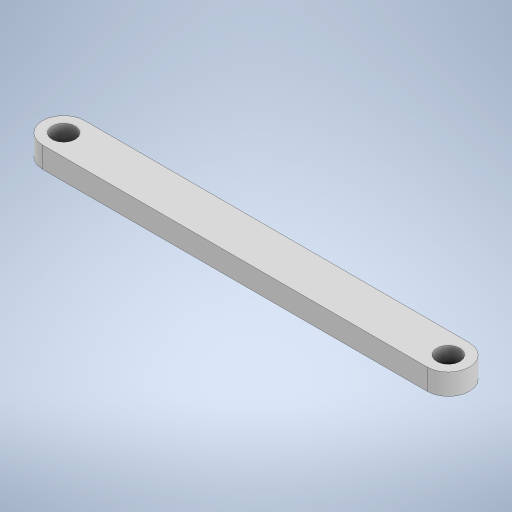
# Autodesk Inventor part: connector
Saved by Autodesk Inventor 2024 (Build 280153000, 153)
## iProperties
Created: 2024-03-19
Part Number: connector
Material: Generic
Document SubType Name: Modeling
Designer: maja6
Density: 1 g/cm^3
Appearance: Default
Author: maja6
Autodesk Inventor part; units mm, degrees
ref_plane "YZ Plane" through (0, 0, 0) normal (1, 0, 0) x (0, 1, 0)
ref_plane "XZ Plane" through (0, 0, 0) normal (0, 1, 0) x (-1, 0, 0)
ref_plane "XY Plane" through (0, 0, 0) normal (0, 0, 1) x (1, 0, 0)
sketch "Sketch1" plane through (0, 0, 0) normal (0, 0, 1) x (1, 0, 0)
  line L0 (0, 0) -> (24, 0)
  circle A0 centre (0, 0) radius 1.6
  line L1 (0, 0) -> (24, 0) construction
  line L2 (0, -3) -> (24, -3)
  line L3 (24, 3) -> (0, 3)
  arc A1 (0, 3) -> (0, -3) centre (0, 0) ccw
  line L4 (24, 0) -> (28, 0)
  circle A2 centre (27, 0) radius 1.6
  line L5 (27, 0) -> (0, 0) construction
  line L6 (27, 3) -> (0, 3)
  line L7 (0, -3) -> (27, -3)
  arc A3 (27, -3) -> (27, 3) centre (27, 0) ccw
  arc A4 (0, 3) -> (0, -3) centre (0, 0) ccw
  point P0 (12, 0)
  point P1 (13.5, 0)
  dimension "d0" = 24
  dimension "d1" = 3.2
  dimension "d6" = 4
  dimension "d7" = 3.2
  dimension "d8" = 6
  constraints: 20 end point, 6 point on circle, 6 tangent, 5 centre point, 3 horizontal, 2 coincident, 2 midpoint, 2 parallel, 1 collinear, 1 point on line
  measures "d0" distance of L0.start L0.end
  measures "d1" diameter of A0
  measures "d6" distance of L1.end L4.end
  measures "d7" diameter of A2
  measures "d8" diameter of A4
extrude "Extrusion1" [suppressed]
sketch "Sketch2" plane through (0, 0, 0) normal (0, 0, 1) x (1, 0, 0)
  line L0 (0, 0) -> (28, 0)
  circle A0 centre (0, 0) radius 1.65
  circle A1 centre (28, 0) radius 1.65
  line L1 (0, 0) -> (28, 0) construction
  line L2 (0, -3) -> (28, -3)
  line L3 (28, 3) -> (0, 3)
  arc A2 (0, 3) -> (0, -3) centre (0, 0) ccw
  arc A3 (28, -3) -> (28, 3) centre (28, 0) ccw
  point P0 (14, 0)
  dimension "d9" = 28
  dimension "d10" = 3.3
  dimension "d11" = 3.3
  dimension "d12" = 6
  constraints: 10 end point, 4 centre point, 4 point on circle, 4 tangent, 2 coincident, 2 equal length, 1 horizontal, 1 midpoint
  measures "d9" distance of L0.start L0.end
  measures "d10" diameter of A0
  measures "d11" diameter of A1
  measures "d12" diameter of A3
extrude "Extrusion2" add sketch "Sketch2" along normal blind 3
sketch "Sketch3" plane through (0, 0, 3) normal (0, 0, 1) x (1, 0, 0)
  circle A0 centre (28, 0) radius 1.65 projected
  line L0 (28, 0) -> (43, 0)
  line L1 (28, 0) -> (43, 0) construction
  line L2 (28, -3) -> (43, -3)
  line L3 (43, 3) -> (28, 3)
  arc A1 (28, 3) -> (28, -3) centre (28, 0) ccw
  arc A2 (43, -3) -> (43, 3) centre (43, 0) ccw
  circle A3 centre (43, 0) radius 1.65
  point P0 (0, 0)
  point P1 (35.5, 0)
  dimension "d15" = 15
  dimension "d16" = 6
  constraints: 10 end point, 4 point on circle, 4 tangent, 3 centre point, 2 equal length, 1 coincident, 1 horizontal, 1 midpoint
  measures "d15" distance of L0.start L0.end
  measures "d16" diameter of A2
extrude "Extrusion3" add sketch "Sketch3" against normal blind 3 contours A0 | A1 L3 A2 L2
sketch "Sketch4" plane through (0, 0, 3) normal (0, 0, 1) x (1, 0, 0)
  line L0 (38.0198, 0) -> (46.7499, 0)
  circle A0 centre (46.7499, 0) radius 1.65
  line L1 (0, 0) -> (46.7499, 0) construction
  line L2 (0, -3) -> (46.7499, -3)
  line L3 (46.7499, 3) -> (0, 3)
  arc A1 (0, 3) -> (0, -3) centre (0, 0) ccw
  arc A2 (46.7499, -3) -> (46.7499, 3) centre (46.7499, 0) ccw
  line L4 (39.9731, -3) -> (39.9731, 3)
  point P0 (23.375, 0)
  dimension "d19" = 3.3
  dimension "d20" = 6
  constraints: 12 end point, 4 point on circle, 4 tangent, 3 centre point, 2 horizontal, 2 point on line, 1 coincident, 1 midpoint, 1 parallel, 1 perpendicular
  measures "d19" diameter of A0
  measures "d20" diameter of A2
extrude "Extrusion4" add sketch "Sketch4" against normal blind 3 contours L4 L3 A2 L2
extrude "Extrusion5" cut sketch "Sketch4" against normal blind 3 contours A0
sketch "Sketch5" plane through (0, 0, 3) normal (0, 0, 1) x (1, 0, 0)
  arc A0 (46.7499, -3) -> (46.7499, 3) centre (46.7499, 0) ccw projected
  line L0 (46.7499, 0) -> (54.7499, 0)
  circle A1 centre (54.7499, 0) radius 1.65
  line L1 (33.9937, 0) -> (54.7499, 0) construction
  line L2 (33.9937, 3) -> (54.7499, 3)
  line L3 (54.7499, -3) -> (33.9937, -3)
  arc A2 (33.9937, 3) -> (33.9937, -3) centre (33.9937, 0) ccw
  arc A3 (54.7499, -3) -> (54.7499, 3) centre (54.7499, 0) ccw
  point P0 (0, 0)
  point P1 (44.3718, 0)
  dimension "d25" = 8
  dimension "d26" = 3.3
  constraints: 10 end point, 4 point on circle, 4 tangent, 3 centre point, 2 horizontal, 1 coincident, 1 midpoint, 1 parallel
  measures "d25" distance of L0.start L0.end
  measures "d26" diameter of A1
extrude "Extrusion6" add sketch "Sketch5" against normal blind 3
body "Solid1"
